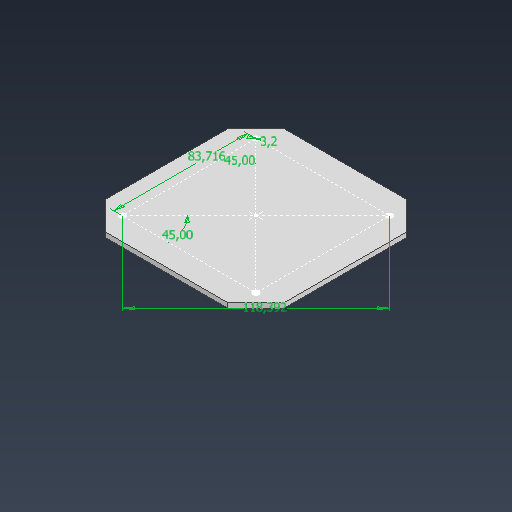
# Autodesk Inventor part: GPS-Compass_top
Saved by Autodesk Inventor 2026.2 (Build 302298000, 298)
## iProperties
Created: 2025-11-17
Part Number: GPS-Compass_top
Material: Generic
Document SubType Name: Modeling
Designer: MenMe
Density: 1 g/cm^3
Appearance: Default
Author: MenMe
Autodesk Inventor part; units mm, degrees
ref_plane "YZ Plane" through (0, 0, 0) normal (1, 0, 0) x (0, 1, 0)
ref_plane "XZ Plane" through (0, 0, 0) normal (0, 1, 0) x (-1, 0, 0)
ref_plane "XY Plane" through (0, 0, 0) normal (0, 0, 1) x (1, 0, 0)
sketch "Sketch2" plane through (0, 0, 0) normal (0, 1, 0) x (-1, 0, 0)
  line L0 (-52.25, 0) -> (52.25, 0) construction
  line L1 (0, 52.25) -> (0, -52.25) construction
  line L2 (52.25, 37.3902) -> (52.25, -37.3902)
  line L3 (52.25, 37.3902) -> (37.3902, 52.25)
  line L4 (37.3902, 52.25) -> (-37.3902, 52.25)
  line L5 (-37.3902, 52.25) -> (-52.25, 37.3902)
  line L6 (-52.25, 37.3902) -> (-52.25, -37.3902)
  line L7 (-52.25, -37.3902) -> (-37.3902, -52.25)
  line L8 (-37.3902, -52.25) -> (37.3902, -52.25)
  line L9 (37.3902, -52.25) -> (52.25, -37.3902)
  line L10 (-56, 0) -> (56, 0) construction
  line L11 (0, 56) -> (0, -56) construction
  line L12 (56, 38.3223) -> (56, -38.3223)
  line L13 (56, 38.3223) -> (38.3223, 56)
  line L14 (38.3223, 56) -> (-38.3223, 56)
  line L15 (-38.3223, 56) -> (-56, 38.3223)
  line L16 (-56, 38.3223) -> (-56, -38.3223)
  line L17 (-56, -38.3223) -> (-38.3223, -56)
  line L18 (-38.3223, -56) -> (38.3223, -56)
  line L19 (38.3223, -56) -> (56, -38.3223)
  point P0 (0, 0)
  point P1 (0, 0)
  point P2 (0, 0)
  point P3 (52.25, 0)
  point P4 (0, 0)
  point P5 (0, 0)
  point P6 (56, 0)
  dimension "d0" = 104.5
  dimension "d1" = 104.5
  dimension "d2" = 135
  dimension "d3" = 135
  dimension "d4" = 135
  dimension "d5" = 21.015
  dimension "d6" = 112
  dimension "d7" = 112
  dimension "d8" = 135
  dimension "d9" = 135
  dimension "d10" = 135
  dimension "d11" = 25
  constraints: 40 end point, 14 midpoint, 4 coincident, 4 horizontal, 4 perpendicular, 4 vertical, 2 parallel
  measures "d0" distance of L0.start L0.end
  measures "d1" distance of L1.start L1.end
  measures "d2" angle of L2 L3
  measures "d3" angle of L2 L9
  measures "d4" angle of L5 L6
  measures "d5" distance of L6.end L7.end
  measures "d6" distance of L10.start L10.end
  measures "d7" distance of L11.start L11.end
  measures "d8" angle of L12 L13
  measures "d9" angle of L12 L19
  measures "d10" angle of L15 L16
  measures "d11" distance of L16.end L17.end
extrude "Extrusion1" add sketch "Sketch2" against normal blind 3 contours L2 L9 L8 L7 L6 L5 L4 L3
extrude "Extrusion2" add sketch "Sketch2" along normal blind 3 contours L2 L9 L8 L7 L6 L5 L4 L3 | L12 L19 L18 L17 L16 L15 L14 L13
sketch "Sketch4" plane through (0, 3, 0) normal (0, 1, 0) x (1, 0, 0)
  line L0 (-41.8579, 41.8579) -> (41.8579, -41.8579) construction
  line L1 (-41.8579, -41.8579) -> (41.8579, 41.8579) construction
  line L2 (41.8579, 41.8579) -> (-41.8579, 41.8579) construction
  line L3 (-41.8579, 41.8579) -> (-41.8579, -41.8579) construction
  line L4 (-41.8579, -41.8579) -> (41.8579, -41.8579) construction
  line L5 (41.8579, -41.8579) -> (41.8579, 41.8579) construction
  circle A0 centre (-41.8579, 41.8579) radius 1.6
  circle A1 centre (41.8579, 41.8579) radius 1.6
  circle A2 centre (-41.8579, -41.8579) radius 1.6
  circle A3 centre (41.8579, -41.8579) radius 1.6
  point P0 (0, 0)
  point P1 (0, 0)
  point P2 (0, 0)
  dimension "d21" = 83.7157
  dimension "d22" = 118.3919
  dimension "d23" = 45
  dimension "d24" = 45
  dimension "d25" = 3.2
  constraints: 12 end point, 6 coincident, 4 centre point, 3 equal length, 3 equal radius, 2 midpoint, 2 perpendicular, 1 horizontal
  measures "d21" distance of L2.end L3.end
  measures "d22" distance of L1.start L1.end
  measures "d23" angle of L4 L1
  measures "d24" angle of L0 L3
  measures "d25" diameter of A0
body "Solid1"
